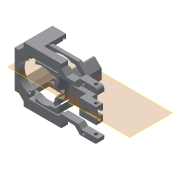
# Autodesk Inventor part: 20_focus_inlet_linearflexure_v0
Saved by Autodesk Inventor 2019.4 (Build 234330000, 330)
## iProperties
Created: 2020-02-03
Part Number: 20_focus_inlet_linearflexure_v0
Material: Generic
Document SubType Name: Modeling
Designer: diederichbenedict
Density: 1 g/cm^3
Appearance: Default
Author: diederichbenedict
Autodesk Inventor part; units mm, degrees
(part 1 of 2)
ref_plane "Work Plane1" through (0, 0, 0) normal (0, 0, 1) x (1, 0, 0)
sketch "Sketch1" plane through (0, 0, 0) normal (0, 0, 1) x (1, 0, 0)
  line L0 (33.5, -15.3849) -> (35.5, -15.3849) projected
  line L1 (35.5, -15.3849) -> (35.5, -14.1603) projected
  arc A0 (35.5, -14.1603) -> (35.3294, -13.8326) centre (35.1, -14.1603) ccw projected
  line L2 (35.3294, -13.8326) -> (34.0923, -12.9664) projected
  arc A1 (33.8775, -12.693) -> (34.0923, -12.9664) centre (34.4364, -12.4749) ccw projected
  arc A2 (33.8775, -12.693) -> (33.8775, -21.107) centre (23.1, -16.9) ccw projected
  arc A3 (34.0923, -20.8336) -> (33.8775, -21.107) centre (34.4364, -21.3251) ccw construction
  line L3 (34.0923, -20.8336) -> (35.3294, -19.9674) construction
  arc A4 (35.3294, -19.9674) -> (35.5, -19.6397) centre (35.1, -19.6397) ccw construction
  line L4 (35.5, -19.6397) -> (35.5, -18.4151) construction
  line L5 (35.5, -18.4151) -> (33.5, -18.4151) construction
  line L6 (33.5, -18.4151) -> (33.5, -15.3849) projected
  line L7 (30.0099, -20.9316) -> (30.0099, -25.4) construction
  line L8 (30.0099, -25.4) -> (27.6057, -25.4) construction
  line L9 (27.6057, -25.4) -> (27.6057, -23.5105) construction
  arc A5 (27.6057, -10.2895) -> (27.6057, -23.5105) centre (23.1, -16.9) ccw construction
  line L10 (27.6057, -10.2895) -> (27.6057, -8.4) construction
  line L11 (27.6057, -8.4) -> (30.0099, -8.4) construction
  line L12 (30.0099, -8.4) -> (30.0099, -12.8684) projected
  arc A6 (30.0099, -20.9316) -> (30.0099, -12.8684) centre (23.1, -16.9) ccw projected
  line L13 (23.1, -16.9) -> (97.1528, -16.9) construction
  arc A7 (31.4223, -8.5777) -> (34.0638, -21.1797) centre (23.1, -16.9) ccw
  arc A8 (34.0638, -12.6203) -> (34.207, -12.8025) centre (34.4364, -12.4749) ccw
  line L14 (34.207, -12.8025) -> (35.4441, -13.6688)
  arc A9 (35.7, -14.1603) -> (35.4441, -13.6688) centre (35.1, -14.1603) ccw
  line L15 (35.7, -14.1603) -> (35.7, -15.5849)
  line L16 (35.7, -15.5849) -> (33.7, -15.5849)
  line L17 (33.7, -15.5849) -> (33.7, -18.2151)
  line L18 (33.7, -18.2151) -> (35.7, -18.2151) construction
  line L19 (35.7, -18.2151) -> (35.7, -19.6397) construction
  arc A10 (35.4441, -20.1312) -> (35.7, -19.6397) centre (35.1, -19.6397) ccw construction
  line L20 (35.4441, -20.1312) -> (34.207, -20.9975) construction
  arc A11 (34.207, -20.9975) -> (34.0638, -21.1797) centre (34.4364, -21.3251) ccw construction
  circle A12 centre (33.6, -15.6849) radius 0.1 construction
  line L21 (35.7, -15.5849) -> (35.7, -16.9) construction
  line L22 (35.7, -15.5849) -> (35.7, -16.9)
  line L23 (23.1, -16.9) -> (31.4223, -8.5777)
  line L24 (23.1, -16.9) -> (34.8695, -16.9) construction
  line L25 (32.6022, -7.3978) -> (33.5436, -6.4564)
  line L26 (33.5436, -6.4564) -> (34.8883, -6.4564)
  line L27 (40.7, -12.2681) -> (40.7, -16.9)
  line L28 (35.7, -16.9) -> (40.7, -16.9)
  line L29 (35.7, -16.9) -> (39.7, -16.9)
  line L30 (39.7, -16.9) -> (39.7, -15.2)
  line L31 (39.7, -15.2) -> (35.7, -15.2)
  line L32 (35.7, -15.2) -> (35.7, -16.9)
  line L33 (39.7, -15.2) -> (36.7, -15.2)
  line L34 (36.7, -15.2) -> (36.7, -13.4)
  line L35 (36.7, -13.4) -> (39.7, -13.4)
  line L36 (39.7, -13.4) -> (39.7, -15.2)
  line L37 (33.5436, -6.4564) -> (34.8883, -6.4564) construction
  line L38 (40.7, -12.2681) -> (34.8883, -6.4564)
  line L39 (40.7, -12.2681) -> (48.919, -12.2681) construction
  arc A13 (34.0638, -12.6203) -> (32.6022, -7.3978) centre (18.0334, -14.2911) ccw
  point P0 (0, 0)
  dimension "d0" = 0.2
  dimension "d1" = 45
  dimension "d2" = 3
  dimension "d6" = 1.7
  dimension "d7" = 4
  dimension "d8" = 3.5
  dimension "d9" = 3
  dimension "d46" = 1
  dimension "d47" = 135
  constraints: 54 end point, 12 point on circle, 7 centre point, 7 horizontal, 4 parallel, 4 perpendicular, 3 point on line, 3 tangent, 2 collinear, 2 equal length, 10 other
  measures "d0" radial gap between concentric circles of A2 A7
  measures "d1" angle of L24 L23
  measures "d2" distance of L23.end L25.end
  measures "d6" distance of L30.end L29.end
  measures "d7" distance between parallel lines of L30 L21
  measures "d8" distance between parallel lines of L13 L35
  measures "d9" distance between parallel lines of L36 L34
  measures "d46" distance between parallel lines of L27 L30
  measures "d47" angle of L39 L38
extrude "Extrusion1" add sketch "Sketch1" against normal blind 35 contours A13 L25 L26 L38 L27 L28 L30 L36 L35 L34 L31 L15 A9 L14 A8
sketch "Sketch2" plane through (0, 0, 0) normal (0, 0, 1) x (1, 0, 0)
  line L0 (39.7, -13.4) -> (39.7, -16.9) projected
  line L1 (39.7, -16.9) -> (40.7, -16.9) projected
  line L2 (40.7, -16.9) -> (40.7, -12.2681) projected
  line L3 (33.5436, -6.4564) -> (32.6022, -7.3978) projected
  arc A0 (34.0638, -12.6203) -> (34.207, -12.8025) centre (34.4364, -12.4749) ccw projected
  line L4 (34.207, -12.8025) -> (35.4441, -13.6688) projected
  arc A1 (35.7, -14.1603) -> (35.4441, -13.6688) centre (35.1, -14.1603) ccw projected
  line L5 (35.7, -14.1603) -> (35.7, -15.2) projected
  line L6 (35.7, -15.2) -> (36.7, -15.2) projected
  line L7 (36.7, -15.2) -> (36.7, -13.4) projected
  line L8 (36.7, -13.4) -> (39.7, -13.4) projected
  line L9 (95.8, 0) -> (0, 0) projected
  line L10 (6, -33.8) -> (89.8, -33.8) projected
  line L11 (6, -33.8) -> (6, 0) projected
  line L12 (11, -0.7) -> (46, -0.7)
  line L13 (45.9987, -4.2) -> (45.9987, -4.7)
  line L14 (11, -4.3971) -> (11, -0.7)
  line L15 (45.9987, -4.7) -> (41.9987, -4.7)
  line L16 (42, -6.1887) -> (42, -16.9)
  line L17 (42, -16.9) -> (46, -16.9)
  line L18 (46, -16.9) -> (46, -10.1887)
  line L19 (6.2, -0.1) -> (10.2, -0.1)
  line L20 (10.2, -0.1) -> (10.2, -16.9)
  line L21 (10.2, -16.9) -> (6.2, -16.9)
  line L22 (6.2, -16.9) -> (6.2, -0.1)
  line L23 (46, -16.9) -> (61, -16.9)
  line L24 (61, -16.9) -> (61, -13.9)
  line L25 (61, -13.9) -> (46, -13.9)
  line L26 (46, -13.9) -> (46, -16.9)
  arc A2 (79.6921, -19.4) -> (79.6921, -14.4) centre (79.6921, -16.9) ccw projected
  line L27 (56, -10.9) -> (56, -13.9)
  line L28 (6.2, -0.1) -> (10.2, -0.1)
  line L29 (10.2, -0.1) -> (10.2, 4.9)
  line L30 (10.2, 4.9) -> (6.2, 4.9)
  line L31 (6.2, 4.9) -> (6.2, -0.1)
  line L32 (1.6162, -33.8) -> (1.6162, 0) projected
  line L33 (-2, 0) -> (1.6162, 0) projected
  line L34 (-2, -33.8) -> (-2, 0) projected
  line L35 (1.6162, -33.8) -> (-2, -33.8) projected
  line L36 (6.2, -16.9) -> (-2, -16.9)
  line L37 (-2, -16.9) -> (-2, -0.2)
  line L38 (-2, -0.2) -> (6.2, -0.2)
  line L39 (6.2, -0.2) -> (6.2, -16.9)
  line L40 (-2, 0) -> (0, 0) projected
  line L41 (10.2, 4.9) -> (89.6, 4.9)
  line L42 (89.6, 4.9) -> (89.6, 0)
  line L43 (89.6, 0) -> (10.2, 0)
  line L44 (10.2, 0) -> (10.2, 4.9)
  line L45 (89.8, 0) -> (89.8, 4.5) projected
  line L46 (95.8, 0) -> (89.8, 0) projected
  line L47 (97.8, -41.8) -> (97.8, 0) construction
  line L48 (94.1838, 0) -> (94.1838, -33.8) projected
  line L49 (97.8, -33.8) -> (94.1838, -33.8) projected
  line L50 (97.8, -33.8) -> (97.8, 0) projected
  line L51 (94.1838, 0) -> (97.8, 0) projected
  line L52 (97.8, -0.2) -> (85.8, -0.2)
  line L53 (85.8, -0.2) -> (85.8, -4.2)
  line L54 (85.8, -4.2) -> (97.8, -4.2)
  line L55 (97.8, -4.2) -> (97.8, -0.2)
  line L56 (85.8, -0.2) -> (89.6, -0.2)
  line L57 (89.6, -0.2) -> (89.6, 0)
  line L58 (89.6, 0) -> (85.8, 0)
  line L59 (85.8, 0) -> (85.8, -0.2)
  line L60 (40.7, -12.2681) -> (34.8883, -6.4564) projected
  line L61 (34.8883, -6.4564) -> (33.5436, -6.4564) projected
  line L62 (42, -12.2664) -> (34.1307, -4.3971)
  line L63 (42, -12.2664) -> (53.1289, -12.2664) construction
  line L64 (36.5113, -0.7) -> (46, -10.1887)
  line L65 (36.5113, -0.7) -> (49.9303, -0.7) construction
  line L66 (45.9987, -4.7) -> (41.9987, -4.7)
  line L67 (34.1307, -4.3971) -> (11, -4.3971)
  line L68 (97.8, -4.2) -> (94.1838, -4.2)
  line L69 (94.1838, -4.2) -> (94.1838, -16.9)
  line L70 (94.1838, -16.9) -> (97.8, -16.9)
  line L71 (97.8, -16.9) -> (97.8, -4.2)
  line L72 (61, -13.9) -> (56, -13.9)
  line L73 (56, -13.9) -> (56, -9.9)
  line L74 (56, -9.9) -> (61, -9.9)
  line L75 (61, -9.9) -> (61, -13.9)
  circle A3 centre (23.1, -16.9) radius 10 projected
  circle A4 centre (23.1, -16.9) radius 12.5 projected
  arc A5 (30.5468, -4.3971) -> (15.6532, -4.3971) centre (23.1, -16.9) ccw
  arc A6 (34.0638, -12.6203) -> (32.6022, -7.3978) centre (18.0334, -14.2911) ccw projected
  dimension "d10" = 35
  dimension "d11" = 4
  dimension "d12" = 5
  dimension "d13" = 0.7
  dimension "d14" = 4
  dimension "d15" = 4
  dimension "d16" = 0.2
  dimension "d17" = 15
  dimension "d18" = 3
  dimension "d25" = 5
  dimension "d28" = 0.1
  dimension "d29" = 5
  dimension "d30" = 0.2
  dimension "d31" = 0.2
  dimension "d32" = 12
  dimension "d33" = 4
  dimension "d34" = 0.2
  dimension "d48" = 135
  dimension "d49" = 45
  dimension "d59" = 1.3
  dimension "d68" = 7
  constraints: 100 end point, 23 parallel, 13 horizontal, 11 perpendicular, 11 point on line, 2 equal length, 2 point on circle, 1 centre point, 1 coincident, 1 midpoint
  measures "d10" distance of L13.end L14.start
  measures "d11" distance of L12.end L13.end
  measures "d12" distance between parallel lines of L14 L11
  measures "d13" distance between parallel lines of L12 L9
  measures "d14" distance of L17.end L16.end
  measures "d15" distance of L20.end L21.end
  measures "d16" distance between parallel lines of L22 L11
  measures "d17" distance of L25.end L24.end
  measures "d18" distance of L24.end L23.end
  measures "d25" distance between parallel lines of L24 L27
  measures "d28" distance between parallel lines of L9 L19
  measures "d29" distance of L29.end L28.end
  measures "d30" distance between parallel lines of L38 L40
  measures "d31" distance between parallel lines of L45 L42
  measures "d32" distance of L54.end L53.end
  measures "d33" distance of L53.end L52.end
  measures "d34" distance between parallel lines of L9 L52
  measures "d48" angle of L63 L62
  measures "d49" angle of L64 L65
  measures "d59" distance between parallel lines of L16 L2
  measures "d68" distance between parallel lines of L74 L23
extrude "Extrusion2" add sketch "Sketch2" against normal blind 6 contours L52 L50 L54 L48 | L48 L54 L53 L52 | L57 L52 L59 L9 | L9 L29 L41 L42 | L54 L50 L70 L48 | L29 L19 L31 L9 | L9 L31 L30 L29 | L20 L21 L22 L19 | L38 L22 L36 L11 | L11 L36 L32 L38 | L32 L36 L34 L38 | L12 L64 L16 L62 L67 A5 L14 | L64 L18 L17 L16 | L25 L24 L23 L18 | L27 L73 L74 L75 L25
sketch "Sketch3" plane through (0, 0, -6) normal (0, 0, 1) x (1, 0, 0)
  line L0 (42, -12.2664) -> (42, -16.9) projected
  line L1 (42, -16.9) -> (61, -16.9) projected
  line L2 (61, -16.9) -> (61, -9.9) projected
  line L3 (56, -13.9) -> (46, -13.9) projected
  line L4 (36.5113, -0.7) -> (11, -0.7) projected
  line L5 (11, -0.7) -> (11, -4.3971) projected
  line L6 (39.7, -13.4) -> (39.7, -16.9) projected
  line L7 (39.7, -16.9) -> (40.7, -16.9) projected
  line L8 (40.7, -16.9) -> (40.7, -12.2681) projected
  line L9 (33.5436, -6.4564) -> (32.6022, -7.3978) projected
  arc A0 (34.0638, -12.6203) -> (34.207, -12.8025) centre (34.4364, -12.4749) ccw projected
  line L10 (34.207, -12.8025) -> (35.4441, -13.6688) projected
  arc A1 (35.7, -14.1603) -> (35.4441, -13.6688) centre (35.1, -14.1603) ccw projected
  line L11 (35.7, -14.1603) -> (35.7, -15.2) projected
  line L12 (35.7, -15.2) -> (36.7, -15.2) projected
  line L13 (36.7, -15.2) -> (36.7, -13.4) projected
  line L14 (36.7, -13.4) -> (39.7, -13.4) projected
  line L15 (6.2, 4.9) -> (6.2, -0.2) projected
  line L16 (-2, -16.9) -> (10.2, -16.9) projected
  line L17 (10.2, -16.9) -> (10.2, 0) projected
  line L18 (11, -4.3971) -> (11, -0.7) projected
  line L19 (10.2, 0) -> (10.2, -16.9) projected
  line L20 (11, -0.7) -> (10.2, -0.7)
  line L21 (10.2, -0.7) -> (10.2, -4.3971)
  line L22 (10.2, -4.3971) -> (11, -4.3971)
  line L23 (11, -4.3971) -> (11, -0.7)
  line L24 (42, -16.9) -> (42, -12.2664) projected
  line L25 (40.7, -16.9) -> (42, -16.9)
  line L26 (42, -16.9) -> (42, -6.4564)
  line L27 (42, -6.4564) -> (40.7, -6.4564)
  line L28 (40.7, -6.4564) -> (40.7, -16.9)
  line L29 (6.2, -0.2) -> (-2, -0.2) projected
  line L30 (-2, -0.2) -> (-2, -16.9) projected
  line L31 (89.6, 4.9) -> (6.2, 4.9) projected
  line L32 (10.2, 0) -> (85.8, 0) projected
  line L33 (89.6, -0.2) -> (89.6, 4.9) projected
  line L34 (85.8, 0) -> (85.8, -4.2) projected
  line L35 (85.8, -4.2) -> (94.1838, -4.2) projected
  line L36 (97.8, -16.9) -> (97.8, -0.2) projected
  line L37 (97.8, -0.2) -> (89.6, -0.2) projected
  line L38 (40.7, -12.2681) -> (34.8883, -6.4564) projected
  line L39 (34.8883, -6.4564) -> (33.5436, -6.4564) projected
  line L40 (46, -13.9) -> (46, -10.1887) projected
  line L41 (46, -10.1887) -> (36.5113, -0.7) projected
  line L42 (30.5468, -4.3971) -> (34.1307, -4.3971) projected
  line L43 (34.1307, -4.3971) -> (42, -12.2664) projected
  line L44 (94.1838, -4.2) -> (94.1838, -16.9) projected
  line L45 (94.1838, -16.9) -> (97.8, -16.9) projected
  line L46 (61, -9.9) -> (56, -9.9) projected
  line L47 (56, -9.9) -> (56, -13.9) projected
  line L48 (11, -4.3971) -> (15.6532, -4.3971) projected
  arc A2 (30.5468, -4.3971) -> (15.6532, -4.3971) centre (23.1, -16.9) ccw projected
  arc A3 (34.0638, -12.6203) -> (32.6022, -7.3978) centre (18.0334, -14.2911) ccw projected
  point P0 (0, 0)
  point P1 (42, -4.4)
  point P2 (10.2, -0.1)
  point P3 (10.2, 4.9)
  constraints: 16 end point, 4 parallel, 2 horizontal, 2 perpendicular, 2 point on line
extrude "Extrusion3" add sketch "Sketch3" along normal blind 0.5 contours L43 L28 L27 L26 | L0 L25 L8 L28 L43 | L22 L17 L20 L5
sketch "Sketch5" plane through (0, 0, -6) normal (0, 0, -1) x (-1, 0, 0)
  line L0 (2, -16.9) -> (2, -0.2) projected
  line L1 (2, -0.2) -> (-6.2, -0.2) projected
  line L2 (-6.2, -0.2) -> (-6.2, 4.9) projected
  line L3 (-6.2, 4.9) -> (-89.6, 4.9) projected
  line L4 (-89.6, 4.9) -> (-89.6, -0.2) projected
  line L5 (-89.6, -0.2) -> (-97.8, -0.2) projected
  line L6 (-97.8, -0.2) -> (-97.8, -16.9) projected
  line L7 (-94.1838, -4.2) -> (-85.8, -4.2) projected
  line L8 (-85.8, -4.2) -> (-85.8, 0) projected
  line L9 (-85.8, 0) -> (-10.2, 0) projected
  line L10 (-10.2, -4.3971) -> (-10.2, -16.9) projected
  line L11 (-10.2, -16.9) -> (2, -16.9) projected
  line L12 (-97.8, -16.9) -> (-94.1838, -16.9) projected
  line L13 (-94.1838, -16.9) -> (-94.1838, -4.2) projected
  line L14 (-10.2, -4.3971) -> (-10.2, -0.7) projected
  arc A0 (-1, -16.9) -> (-10.2, -4.3971) centre (-14.0958, -16.9) ccw
  line L15 (-10.2, 0) -> (-10.2, -0.7) projected
  line L16 (-36.5113, -0.7) -> (-10.2, -0.7) projected
  line L17 (-36.5113, -0.7) -> (-46, -10.1887) projected
  line L18 (-46, -10.1887) -> (-46, -13.9) projected
  line L19 (-46, -13.9) -> (-56, -13.9) projected
  line L20 (-56, -13.9) -> (-56, -9.9) projected
  line L21 (-56, -9.9) -> (-61, -9.9) projected
  line L22 (-61, -9.9) -> (-61, -16.9) projected
  line L23 (-61, -16.9) -> (-40.7, -16.9) projected
  line L24 (-40.7, -12.2681) -> (-40.7, -16.9) projected
  line L25 (-40.7, -10.9664) -> (-40.7, -12.2681) projected
  line L26 (-40.7, -10.9664) -> (-34.1307, -4.3971) projected
  line L27 (-34.1307, -4.3971) -> (-30.5468, -4.3971) projected
  arc A1 (-15.6532, -4.3971) -> (-30.5468, -4.3971) centre (-23.1, -16.9) ccw projected
  line L28 (-15.6532, -4.3971) -> (-10.2, -4.3971) projected
  dimension "d65" = 0
  dimension "d66" = 3
  constraints: 2 point on circle, 1 centre point, 1 point on line
  measures "d65" distance from line of A0.centre L11
  measures "d66" distance from line of L0 A0.start
extrude "Extrusion5" cut sketch "Sketch5" against normal through all contours L11 L10 A0
sketch "Sketch6" plane through (0, 0, -6) normal (0, 0, -1) x (-1, 0, 0)
  line L0 (-46, -13.9) -> (-56, -13.9) projected
  line L1 (-61, -9.9) -> (-61, -16.9) projected
  line L2 (-10.2, -16.9) -> (2, -16.9) construction
  line L3 (-10.2, -4.3971) -> (-10.2, -16.9) projected
  line L4 (2, -0.2) -> (2, -16.9) projected
  line L5 (2, -0.2) -> (-10.2, -0.2)
  line L6 (2, -4.4) -> (2, -0.2)
  line L7 (2, -4.4) -> (2, -0.2) construction
  line L8 (2, -0.2) -> (-10.2, -0.2) construction
  line L9 (-36.5113, -0.7) -> (-46, -10.1887) projected
  line L10 (-46, -10.1887) -> (-46, -13.9) projected
  line L11 (-40.7, -10.9664) -> (-34.1307, -4.3971) projected
  line L12 (-56, -13.9) -> (-56, -9.9) projected
  line L13 (-56, -9.9) -> (-61, -9.9) projected
  line L14 (2, -4.4) -> (-10.2, -4.4)
  line L15 (-10.2, -4.4) -> (-10.2, -0.2)
  line L16 (-10.2, -0.2) -> (2, -0.2)
  line L17 (2, -0.2) -> (2, -4.4)
  line L18 (-34.1307, -4.3971) -> (-30.5468, -4.3971) projected
  arc A0 (-15.6532, -4.3971) -> (-30.5468, -4.3971) centre (-23.1, -16.9) ccw projected
  line L19 (-40.7, -10.9664) -> (-40.7, -12.2681) projected
  line L20 (-36.5113, -0.7) -> (-10.2, -0.7) projected
  line L21 (-61, -16.9) -> (-40.7, -16.9) projected
  line L22 (-40.7, -12.2681) -> (-40.7, -16.9) projected
  line L23 (-15.6532, -4.3971) -> (-10.2, -4.3971) projected
  line L24 (2, -16.9) -> (2, -0.2) projected
  line L25 (2, -0.2) -> (-6.2, -0.2) projected
  line L26 (-6.2, -0.2) -> (-6.2, 4.9) projected
  line L27 (-6.2, 4.9) -> (-89.6, 4.9) projected
  line L28 (-89.6, 4.9) -> (-89.6, -0.2) projected
  line L29 (-89.6, -0.2) -> (-97.8, -0.2) projected
  line L30 (-97.8, -0.2) -> (-97.8, -16.9) projected
  line L31 (-97.8, -16.9) -> (-94.1838, -16.9) projected
  line L32 (-94.1838, -16.9) -> (-94.1838, -4.2) projected
  line L33 (-94.1838, -4.2) -> (-85.8, -4.2) projected
  line L34 (-85.8, -4.2) -> (-85.8, 0) projected
  line L35 (-85.8, 0) -> (-10.2, 0) projected
  line L36 (-10.2, 0) -> (-10.2, -0.7) projected
  line L37 (-10.2, -4.3971) -> (-10.2, -16.9) projected
  line L38 (-10.2, -16.9) -> (2, -16.9) projected
  line L39 (2, -16.9) -> (2, -0.2) projected
  line L40 (2, -0.2) -> (-6.2, -0.2) projected
  line L41 (-6.2, -0.2) -> (-6.2, 4.9) projected
  line L42 (-6.2, 4.9) -> (-89.6, 4.9) projected
  line L43 (-89.6, 4.9) -> (-89.6, -0.2) projected
  line L44 (-89.6, -0.2) -> (-97.8, -0.2) projected
  line L45 (-97.8, -0.2) -> (-97.8, -16.9) projected
  line L46 (-97.8, -16.9) -> (-94.1838, -16.9) projected
  line L47 (-94.1838, -16.9) -> (-94.1838, -4.2) projected
  line L48 (-94.1838, -4.2) -> (-85.8, -4.2) projected
  line L49 (-85.8, -4.2) -> (-85.8, 0) projected
  line L50 (-85.8, 0) -> (-10.2, 0) projected
  line L51 (-10.2, 0) -> (-10.2, -0.7) projected
  line L52 (-36.5113, -0.7) -> (-10.2, -0.7) projected
  line L53 (-36.5113, -0.7) -> (-46, -10.1887) projected
  line L54 (-46, -10.1887) -> (-46, -13.9) projected
  line L55 (-46, -13.9) -> (-56, -13.9) projected
  line L56 (-56, -13.9) -> (-56, -9.9) projected
  line L57 (-56, -9.9) -> (-61, -9.9) projected
  line L58 (-61, -9.9) -> (-61, -16.9) projected
  line L59 (-61, -16.9) -> (-40.7, -16.9) projected
  line L60 (-40.7, -12.2681) -> (-40.7, -16.9) projected
  line L61 (-40.7, -10.9664) -> (-40.7, -12.2681) projected
  line L62 (-40.7, -10.9664) -> (-34.1307, -4.3971) projected
  line L63 (-34.1307, -4.3971) -> (-30.5468, -4.3971) projected
  arc A1 (-15.6532, -4.3971) -> (-30.5468, -4.3971) centre (-23.1, -16.9) ccw projected
  line L64 (-15.6532, -4.3971) -> (-10.2, -4.3971) projected
  point P0 (0, 0)
  constraints: 16 end point, 2 horizontal, 2 parallel, 1 perpendicular
ref_plane "Work Plane2" through (6, 4.5, -33.8) normal (0, 0, 1) x (1, 0, 0)
extrude "Extrusion6" add sketch "Sketch6" along normal up to surface (27.8 mm away) contours L15 L5 L4 L14 L3
ref_plane "Work Plane3" through (0, 0, -18) normal (0, 0, -1) x (-1, 0, 0)
sketch "Sketch7" plane through (0, 0, -18) normal (0, 0, -1) x (-1, 0, 0)
  line L0 (-11, -0.7) -> (-10.2, -0.7) projected
  line L1 (-10.2, -4.3971) -> (-11, -4.3971) projected
  line L2 (-11.9304, -0.7) -> (-11, -0.7) projected
  line L3 (-11.9304, -4.3971) -> (-11.9304, -0.7) projected
  line L4 (-46, -13.9) -> (-56, -13.9) projected
  line L5 (-61, -9.9) -> (-61, -16.9) projected
  line L6 (-40.7, -16.9) -> (-42, -16.9) projected
  line L7 (-40.7, -16.9) -> (-40.7, -12.2681) projected
  line L8 (-10.2, -0.2) -> (-10.2, -4.4) projected
  line L9 (2, -4.4) -> (2, -0.2) projected
  line L10 (2, -0.2) -> (-10.2, -0.2) projected
  line L11 (-46, -13.9) -> (-46, -16.9)
  line L12 (-61, -16.9) -> (-42, -16.9) projected
  line L13 (-40.7, -10.9664) -> (-40.7, -12.2681) projected
  line L14 (-36.5113, -0.7) -> (-46, -10.1887) projected
  line L15 (-46, -10.1887) -> (-46, -13.9) projected
  line L16 (-40.7, -10.9664) -> (-34.1307, -4.3971) projected
  line L17 (-11, -4.3971) -> (-11.9304, -4.3971) projected
  line L18 (-46, -13.9) -> (-46, -16.9)
  line L19 (-56, -13.9) -> (-56, -9.9) projected
  line L20 (-56, -9.9) -> (-61, -9.9) projected
  line L21 (-10.2, -4.4) -> (2, -4.4) projected
  line L22 (-34.1307, -4.3971) -> (-30.5468, -4.3971) projected
  arc A0 (-15.6532, -4.3971) -> (-30.5468, -4.3971) centre (-23.1, -16.9) ccw projected
  line L23 (-11, -0.7) -> (-11, -4.3971) projected
  line L24 (-40.7, -10.9664) -> (-40.7, -12.2681) projected
  line L25 (-40.7, -10.9664) -> (-42, -12.2664) projected
  line L26 (-42, -12.2664) -> (-42, -16.9) projected
  line L27 (-36.5113, -0.7) -> (-10.2, -0.7) projected
  line L28 (-61, -16.9) -> (-40.7, -16.9) projected
  line L29 (-40.7, -12.2681) -> (-40.7, -16.9) projected
  line L30 (-15.6532, -4.3971) -> (-10.2, -4.3971) projected
  line L31 (-11, -0.7) -> (-11, -4.3971) projected
  line L32 (-10.2, -4.3971) -> (-10.2, -0.7) projected
  line L33 (-10.2, -4.3971) -> (-10.2, -0.7) projected
  point P0 (0, 0)
  constraints: 4 end point, 1 collinear, 1 point on line
extrude "Extrusion7" add sketch "Sketch7" along normal blind 3 contours L23 L17 L3 L2 | L3 L30 A0 L22 L16 L25 L26 L12 L11 L15 L14 L27
sketch "Sketch8" plane through (0, 0, -18) normal (0, 0, 1) x (1, 0, 0)
  line L0 (11, -0.7) -> (10.2, -0.7) projected
  line L1 (10.2, -4.3971) -> (11, -4.3971) projected
  line L2 (40.7, -16.9) -> (42, -16.9) projected
  line L3 (40.7, -16.9) -> (40.7, -12.2681) projected
  line L4 (40.7, -10.9664) -> (40.7, -12.2681) projected
  line L5 (40.7, -10.9664) -> (42, -12.2664) projected
  line L6 (42, -12.2664) -> (42, -16.9) projected
  line L7 (11, -0.7) -> (11, -4.3971) projected
  line L8 (10.2, -4.3971) -> (10.2, -0.7) projected
  point P0 (0, 0)
  point P1 (10.2, -4.4)
extrude "Extrusion8" add sketch "Sketch8" against normal blind 0.5
sketch "Sketch9" plane through (10.2, -0.7, -18) normal (0, 1, 0) x (1, 0, 0)
  line L0 (26.3113, 0) -> (0, 0) projected
  line L1 (26.3113, 0) -> (26.3113, 3) projected
  line L2 (0, 3) -> (26.3113, 3) projected
  line L3 (0, 0) -> (0, 3) projected
  line L4 (0.8, 0.5) -> (0, 0.5) projected
  line L5 (0.8, 0.5) -> (1.8167, 3)
  line L6 (23.9307, 3) -> (0.8, 3) projected
  line L7 (0.8, 3) -> (1.8167, 3)
  line L8 (0.8, 3) -> (0.8, 0.5)
  point P0 (-10.2, -18)
  constraints: 6 end point, 1 collinear, 1 point on line
extrude "Extrusion9" cut sketch "Sketch9" against normal up to surface (3.6971 mm away) contours L8 L2 L5
sketch "Sketch10" plane through (0, 0, -6) normal (0, 0, -1) x (-1, 0, 0)
  arc A0 (-75.8, -1.5) -> (-75.8, 2.7) centre (-75.8, 0.6) ccw projected
  line L0 (-10.2, 0) -> (-10.2, -0.2) projected
  line L1 (-89.6, 4.9) -> (-72.3075, 4.9)
  line L2 (-72.3075, 4.9) -> (-72.3075, -2.4765)
  line L3 (-72.3075, -2.4765) -> (-89.6, -2.4765)
  line L4 (-89.6, -2.4765) -> (-89.6, 4.9)
  line L5 (-10.2, -16.9) -> (2, -16.9) projected
  line L6 (2, -4.4) -> (-10.2, -4.4) projected
  line L7 (-10.2, -0.2) -> (-6.2, -0.2) projected
  line L8 (-6.2, -0.2) -> (-6.2, 4.9) projected
  line L9 (-6.2, 4.9) -> (-89.6, 4.9) projected
  line L10 (-89.6, 4.9) -> (-89.6, -0.2) projected
  line L11 (-89.6, -0.2) -> (-97.8, -0.2) projected
  line L12 (-97.8, -0.2) -> (-97.8, -16.9) projected
  line L13 (-97.8, -16.9) -> (-94.1838, -16.9) projected
  line L14 (-94.1838, -16.9) -> (-94.1838, -4.2) projected
  line L15 (-94.1838, -4.2) -> (-85.8, -4.2) projected
  line L16 (-85.8, -4.2) -> (-85.8, 0) projected
  line L17 (-85.8, 0) -> (-10.2, 0) projected
  line L18 (-10.2, -4.4) -> (-10.2, -16.9) projected
  line L19 (2, -16.9) -> (2, -4.4) projected
  point P0 (0, 0)
  constraints: 8 end point, 2 parallel, 1 horizontal, 1 perpendicular
ref_plane "Work Plane4" through (10.2, -4.4, -20.3) normal (0, 0, -1) x (-1, 0, 0)
extrude "Extrusion10" add sketch "Sketch10" along normal up to surface (14.3 mm away) contours L17 L16 L3 L4 L1 L2 | L2 L3 L16 L17
sketch "Sketch11" plane through (89.6, 4.9, -20.3) normal (0, 0, -1) x (-1, 0, 0)
  arc A0 (13.8, -6.4) -> (13.8, -2.2) centre (13.8, -4.3) ccw projected
  circle A1 centre (13.8, -4.3) radius 1.4
  point P0 (89.6, -4.9)
  dimension "d54" = 2.8
  constraints: 1 centre point, 1 coincident
  measures "d54" diameter of A1
extrude "Extrusion11" cut sketch "Sketch11" against normal through all
sketch "Sketch13" plane through (61, -16.9, 0) normal (1, 0, 0) x (0, 0, -1)
  line L0 (0, 3) -> (6, 3) projected
  line L1 (6, 0) -> (6, 4.6336) projected
  line L2 (0, 0) -> (35, 0) projected
  line L3 (21, 0) -> (18, 0) projected
  line L4 (0, 4.6319) -> (0, 10.4436) projected
  line L5 (0, 10.4436) -> (0, 9.5022) projected
  line L6 (0, 4.2797) -> (0, 4.0975) projected
  line L7 (0, 4.0975) -> (0, 3.2312) projected
  line L8 (0, 3.2312) -> (0, 2.7397) projected
  line L9 (0, 2.7397) -> (0, 1.7) projected
  line L10 (0, 1.7) -> (0, 3.5) projected
  line L11 (0, 3.5) -> (0, 0) projected
  line L12 (0, 0) -> (6, 0) projected
  line L13 (6, 0) -> (0, 0)
  line L14 (0, 0) -> (0, 1.7)
  line L15 (0, 1.7) -> (6, 1.7)
  line L16 (6, 1.7) -> (6, 0)
  line L17 (35, 1.7) -> (0, 1.7) projected
  line L18 (4.864, 1.7) -> (1.364, 1.7)
  line L19 (1.364, 1.7) -> (1.364, 4.55)
  line L20 (1.364, 4.55) -> (4.864, 4.55)
  line L21 (4.864, 4.55) -> (4.864, 1.7)
  line L22 (6, 1.7) -> (4.364, 1.7)
  line L23 (4.364, 1.7) -> (4.364, 7)
  line L24 (4.364, 7) -> (6, 7)
  line L25 (6, 7) -> (6, 1.7)
  line L26 (1.364, 4.55) -> (4.364, 4.55)
  line L27 (4.364, 4.55) -> (4.364, 7)
  line L28 (4.364, 7) -> (1.364, 7)
  line L29 (1.364, 7) -> (1.364, 4.55)
  line L30 (1.364, 7) -> (0, 7)
  line L31 (0, 7) -> (0, 1.7)
  line L32 (0, 1.7) -> (1.364, 1.7)
  line L33 (1.364, 1.7) -> (1.364, 7)
  line L34 (0, 3) -> (6, 3) projected
  line L35 (0, 9.5022) -> (0, 4.2797) projected
  line L36 (0, 0) -> (0, 4.6319) projected
  line L37 (18.5, 0) -> (35, 0) projected
  line L38 (6, 0) -> (18, 0) projected
  line L39 (0, 0) -> (6, 0) projected
  line L40 (0, 0) -> (5.5, 0) projected
  line L41 (0, 0) -> (5.5, 0) projected
  line L42 (18.5, 0) -> (21, 0) projected
  point P0 (0, 16.9)
  point P1 (6, 3)
  point P2 (6.5, 0)
  point P3 (0.5, 0)
  point P4 (0, 0)
  point P5 (0, 0)
  point P6 (0, 0)
  point P7 (0, 18.6)
  point P8 (0, 21.4)
  point P9 (0, 18.6)
  point P10 (0, 21.4)
  dimension "d60" = 1.7
  dimension "d61" = 3.5
  dimension "d62" = 2.85
  constraints: 40 end point, 10 parallel, 5 horizontal, 5 perpendicular, 1 point on line, 1 other
  measures "d60" distance of L13.end L10.start
  measures "d61" distance of L19.end L20.end
  measures "d62" distance of L18.end L19.end
extrude "Extrusion13" add sketch "Sketch13" along normal blind 10 contours L8 L7 L6 L31 L4 L30 L29 L19 L0 | L0 L19 L15 L9 L8 | L23 L20 L21 L0 | L0 L21 L15 L23 | L29 L28 L23 L20 | L21 L20 L23 L24 L25 L1 L0 | L0 L1 L15 L21
mirror "Mirror1" about plane through (6.2, -16.9, 0) normal (0, -1, 0) of "Extrusion1", "Extrusion2", "Extrusion3", "Extrusion5", "Extrusion6", "Extrusion7", "Extrusion8", "Extrusion9", "Extrusion10", "Extrusion11", "Extrusion13"
sketch "Sketch14" plane through (56, -9.9, 0) normal (0, 1, 0) x (1, 0, 0)
  line L0 (9.3, 20.8) -> (9.3, 18.3)
  line L1 (33.6, 0) -> (-49.8, 0) projected
  line L2 (33.6, 0) -> (33.6, 20.3) projected
  line L3 (33.6, 20.3) -> (16.3075, 20.3) projected
  line L4 (16.3075, 6) -> (16.3075, 20.3) projected
  line L5 (-49.8, 6) -> (16.3075, 6) projected
  line L6 (-49.8, 0) -> (-49.8, 6) projected
  circle A0 centre (11.813, 3) radius 1.45
  point P0 (-56, 0)
  point P1 (14.3156, 19.0518)
  dimension "d69" = 2.9
  constraints: 2 end point, 1 centre point, 1 vertical, 3 other
  measures "d69" diameter of A0
extrude "Extrusion14" cut sketch "Sketch14" along normal through all both and the other way through all contours A0
sketch "Sketch15" plane through (89.6, 4.9, -20.3) normal (0, 0, -1) x (-1, 0, 0)
  circle A0 centre (13.8, -4.3) radius 1.4 projected
  line L0 (0, 0) -> (17.2925, 0) projected
  line L1 (0, -7.3765) -> (0, 0) projected
  line L2 (17.2925, -7.3765) -> (0, -7.3765) projected
  line L3 (17.2925, 0) -> (17.2925, -7.3765) projected
  line L4 (-0.2, -38.7) -> (83.6, -38.7) projected
  circle A1 centre (13.8, -39.3) radius 1.4 projected
  line L5 (0, -43.6) -> (17.2925, -43.6) projected
  line L6 (17.2925, -43.6) -> (17.2925, -36.2235) projected
  line L7 (17.2925, -36.2235) -> (0, -36.2235) projected
  line L8 (0, -36.2235) -> (0, -43.6) projected
  line L9 (0, -36.2235) -> (3.8, -36.2235) projected
  line L10 (0, -43.6) -> (17.2925, -43.6) projected
  line L11 (0, -36.2235) -> (6, -36.2235)
  line L12 (6, -36.2235) -> (6, -43.6)
  line L13 (6, -43.6) -> (0, -43.6)
  line L14 (0, -43.6) -> (0, -36.2235)
  line L15 (0, 0) -> (17.2925, 0) projected
  line L16 (0, -7.3765) -> (6, -7.3765)
  line L17 (6, -7.3765) -> (6, 0)
  line L18 (6, 0) -> (0, 0)
  line L19 (0, 0) -> (0, -7.3765)
  point P0 (89.6, -4.9)
  dimension "d72" = 6
  constraints: 16 end point, 4 parallel, 3 point on line, 2 horizontal, 2 perpendicular
  measures "d72" distance of L12.end L13.end
extrude "Extrusion15" add sketch "Sketch15" along normal up to surface (13.5 mm away) contours L0 L17 L2 L1 | L8 L7 L12 L4 | L4 L12 L5 L8
sketch "Sketch16" plane through (0, 0, -6) normal (0, 0, -1) x (-1, 0, 0)
  line L0 (-10.1907, -29.4) -> (2, -29.4) construction
  line L1 (2, -4.4) -> (-10.1907, -4.4) construction
  line L2 (-10.1907, -4.4) -> (2, -4.4)
  line L3 (-10.1907, -29.4) -> (2, -29.4)
  line L4 (2, -29.4) -> (2, -27.4)
  line L5 (2, -33.6) -> (2, -33.6) projected
  line L6 (2, -27.4) -> (-6.2696, -27.4)
  arc A0 (-10.2, -29.4029) -> (-10.2, -4.3971) centre (-14.0958, -16.9) ccw projected
  line L7 (2, -4.4) -> (2, -6.4)
  line L8 (2, -6.4) -> (-6.2696, -6.4)
  arc A1 (-10.1907, -29.4) -> (-6.2696, -27.4) centre (-14.0958, -16.9) ccw
  arc A2 (-6.2696, -6.4) -> (-10.1907, -4.4) centre (-14.0958, -16.9) ccw
  line L9 (-10.2, -4.3971) -> (-10.2, -0.7) projected
  line L10 (2, -4.4) -> (2, -29.4) projected
  line L11 (-72.3075, 4.9) -> (-72.3075, 0) projected
  line L12 (-72.3075, 0) -> (-10.2, 0) projected
  line L13 (-10.2, 0) -> (-10.2, -0.2) projected
  line L14 (-10.2, -0.2) -> (-6.2, -0.2) projected
  line L15 (-6.2, -0.2) -> (-6.2, 4.9) projected
  line L16 (-6.2, 4.9) -> (-72.3075, 4.9) projected
  arc A3 (-10.1907, -29.4) -> (-10.1907, -4.4) centre (-14.0958, -16.9) ccw projected
  line L17 (-10.2, -33.1) -> (-10.2, -29.4029) projected
  line L18 (-10.2, -29.4029) -> (-15.6532, -29.4029) projected
  arc A4 (-15.6532, -29.4029) -> (-30.5468, -29.4029) centre (-23.1, -16.9) ccw projected
  line L19 (-34.1307, -29.4029) -> (-30.5468, -29.4029) projected
  line L20 (-40.7, -22.8336) -> (-34.1307, -29.4029) projected
  line L21 (-40.7, -22.8336) -> (-40.7, -21.5319) projected
  line L22 (-40.7, -12.2681) -> (-40.7, -21.5319) projected
  line L23 (-40.7, -10.9664) -> (-40.7, -12.2681) projected
  line L24 (-40.7, -10.9664) -> (-34.1307, -4.3971) projected
  line L25 (-34.1307, -4.3971) -> (-30.5468, -4.3971) projected
  arc A5 (-15.6532, -4.3971) -> (-30.5468, -4.3971) centre (-23.1, -16.9) ccw projected
  line L26 (-15.6532, -4.3971) -> (-10.2, -4.3971) projected
  line L27 (-36.5113, -0.7) -> (-10.2, -0.7) projected
  line L28 (-36.5113, -0.7) -> (-46, -10.1887) projected
  line L29 (-46, -10.1887) -> (-46, -13.9) projected
  line L30 (-46, -13.9) -> (-56, -13.9) projected
  line L31 (-56, -13.9) -> (-56, -9.9) projected
  line L32 (-56, -9.9) -> (-71, -9.9) projected
  line L33 (-71, -15.2) -> (-71, -9.9) projected
  line L34 (-61, -15.2) -> (-71, -15.2) projected
  line L35 (-61, -15.2) -> (-61, -18.6) projected
  line L36 (-61, -18.6) -> (-71, -18.6) projected
  line L37 (-71, -18.6) -> (-71, -23.9) projected
  line L38 (-56, -23.9) -> (-71, -23.9) projected
  line L39 (-56, -19.9) -> (-56, -23.9) projected
  line L40 (-46, -19.9) -> (-56, -19.9) projected
  line L41 (-46, -23.6113) -> (-46, -19.9) projected
  line L42 (-36.5113, -33.1) -> (-46, -23.6113) projected
  line L43 (-10.2, -33.1) -> (-36.5113, -33.1) projected
  line L44 (-72.3075, -33.8) -> (-72.3075, -38.7) projected
  line L45 (-6.2, -38.7) -> (-72.3075, -38.7) projected
  line L46 (-6.2, -33.6) -> (-6.2, -38.7) projected
  line L47 (-6.2, -33.6) -> (-10.2, -33.6) projected
  line L48 (-10.2, -33.8) -> (-10.2, -33.6) projected
  line L49 (-72.3075, -33.8) -> (-10.2, -33.8) projected
  point P0 (0, 0)
  point P1 (2, -0.2)
  dimension "d76" = 2
  dimension "d77" = 2
  constraints: 12 end point, 5 point on circle, 2 centre point, 2 concentric, 2 perpendicular, 2 other
  measures "d76" distance of L3.end L4.end
  measures "d77" distance of L2.end L7.end
extrude "Extrusion16" add sketch "Sketch16" along normal up to surface (27.8 mm away) contours L2 L7 L8 A0 | L6 L4 L3 A0
sketch "Sketch17" plane through (-2, -0.2, -33.8) normal (-1, 0, 0) x (0, 0, 1)
  line L0 (33.8, 0) -> (0, 0) construction
  line L1 (0, -6.2) -> (0, 0) construction
  line L2 (27.8, -6.2) -> (0, -6.2) construction
  line L3 (27.8, -6.2) -> (27.8, -27.2) construction
  line L4 (27.8, -27.2) -> (0, -27.2) construction
  line L5 (0, -27.2) -> (0, -33.4) construction
  line L6 (33.8, -33.4) -> (0, -33.4) construction
  line L7 (32.15, -3.5) -> (1.65, -3.5) construction
  line L8 (1.65, -3.5) -> (1.65, -29.9) construction
  line L9 (1.65, -29.9) -> (32.15, -29.9) construction
  line L10 (32.15, -29.9) -> (32.15, -3.5) construction
  line L11 (32.15, -3.5) -> (1.65, -29.9) construction
  line L12 (1.65, -3.5) -> (32.15, -29.9) construction
  circle A0 centre (1.65, -29.9) radius 1.5 construction
  circle A1 centre (1.65, -3.5) radius 1.5 construction
  circle A2 centre (32.15, -3.5) radius 1.5 construction
  circle A3 centre (32.15, -29.9) radius 1.5 construction
  circle A4 centre (1.65, -29.9) radius 1.2
  circle A5 centre (1.65, -3.5) radius 1.2
  circle A6 centre (32.15, -29.9) radius 1.2
  circle A7 centre (32.15, -3.5) radius 1.2
  line L13 (33.8, 0) -> (33.8, -33.4) projected
  point P0 (33.8, 0.2)
  point P1 (16.9, -16.7)
  dimension "d80" = 30.5
  dimension "d81" = 26.4
  dimension "d82" = 3
  dimension "d83" = 3
  dimension "d84" = 3
  dimension "d85" = 3
  dimension "d89" = 0.3
  dimension "d90" = 0.3
  dimension "d91" = 0.3
  dimension "d92" = 0.3
  constraints: 12 end point, 8 centre point, 4 coincident, 2 midpoint, 2 parallel, 1 horizontal, 1 perpendicular
  measures "d80" distance of L9.end L8.end
  measures "d81" distance of L8.end L7.end
  measures "d82" diameter of A0
  measures "d83" diameter of A1
  measures "d84" diameter of A2
  measures "d85" diameter of A3
  measures "d89" radial gap between concentric circles of A0 A4
  measures "d90" radial gap between concentric circles of A1 A5
  measures "d91" radial gap between concentric circles of A3 A6
  measures "d92" radial gap between concentric circles of A2 A7
extrude "Extrusion17" cut sketch "Sketch17" against normal up to surface (12.2 mm away)
sketch "Sketch18" plane through (0, 0, -6) normal (0, 0, -1) x (-1, 0, 0)
  line L0 (-39.8, 8) -> (-39.8, 4.3838) projected
  line L1 (-44.1838, 0) -> (-47.8, 0) projected
  line L2 (-47.8, 6) -> (-47.8, -39.8) projected
  circle A0 centre (-42.9, 3.1) radius 3 projected
  line L3 (-6.2, 4.9) -> (-72.3075, 4.9) projected
  line L4 (-39.7, 4.9) -> (-39.7, 0)
  line L5 (-72.3075, 0) -> (-10.2, 0) projected
  line L6 (-39.7, 4.9) -> (-47.9, 4.9)
  line L7 (-47.9, 4.9) -> (-47.9, -0.1)
  line L8 (-47.9, -0.1) -> (-39.7, -0.1)
  line L9 (-39.7, -0.1) -> (-39.7, 4.9)
  line L10 (-47.9, -0.1) -> (-55.9, -0.1)
  line L11 (-55.9, -0.1) -> (-55.9, 4.9)
  circle A1 centre (-52.7, 3.1) radius 1.1933 projected
  circle A2 centre (-52.7, 3.1) radius 1.4 projected
  circle A3 centre (-52.7, 3.1) radius 1.6 projected
  circle A4 centre (-52.7, 3.1) radius 1.5 projected
  circle A5 centre (-52.7, 3.1) radius 2.75 projected
  circle A6 centre (-52.7, 3.1) radius 1.4 projected
  point P0 (0, 0)
  dimension "d95" = 0.1
  dimension "d97" = 0.1
  dimension "d98" = 0.1
  dimension "d107" = 3.2
  constraints: 14 end point, 3 point on line, 2 horizontal, 2 parallel, 2 perpendicular, 1 vertical
  measures "d95" distance between parallel lines of L4 L0
  measures "d97" distance between parallel lines of L5 L8
  measures "d98" distance between parallel lines of L7 L2
  measures "d107" distance from line of L11 A3.centre
extrude "Extrusion18" cut sketch "Sketch18" against normal up to surface (6 mm away) contours L5 L9 L8 L2 L1 | L1 L2 L3 A0 L4 L5 | L5 L7 L3 L2 | L2 L8 L7 L5 | L7 L10 L11 L5 | L5 L11 L3 A5 L7 | L3 A0 | A5 L3 | L3 A5 | A1 | A2 | A3 | A4 picked at (-42.9851, 3.3036)
sketch "Sketch19" plane through (0, 0, -6) normal (0, 0, -1) x (-1, 0, 0)
  line L0 (-42.386, 1.7978) -> (-44.1838, 0) projected
  line L1 (-39.8, 4.3838) -> (-41.5978, 2.586) projected
  line L2 (-47.8, 6) -> (-47.8, -39.8) projected
  line L3 (-72.3075, 0) -> (-10.2, 0) projected
  line L4 (-39.7, 0) -> (-39.7, 4.9) projected
  line L5 (-44.1019, -0.0818) -> (-47.9, -0.0818)
  line L6 (-47.9, -0.0818) -> (-47.9, 0)
  line L7 (-54.7, 0) -> (-39.7, 0)
  line L8 (-39.7, 0) -> (-39.7, -3)
  line L9 (-39.7, -3) -> (-54.7, -3)
  line L10 (-54.7, -3) -> (-54.7, 0)
  line L11 (-39.7, -3) -> (-36.7, 0)
  line L12 (-39.7, -3) -> (-35.4574, -3) construction
  line L13 (-39.7, 0) -> (-36.7, 0)
  line L14 (-39.7, 0) -> (-10.2, 0) projected
  line L15 (-54.7, -3) -> (-57.7, 0)
  line L16 (-54.7, -3) -> (-50.4574, -3) construction
  line L17 (-57.7, 0) -> (-54.7, 0)
  line L18 (-47.9, -0.0818) -> (-51.4981, -0.0818)
  line L19 (-55.9, 4.9) -> (-55.9, 0) projected
  line L20 (-55.9, 4.3201) -> (-55.9, 0)
  line L21 (-57.7, 0) -> (-55.9, 0)
  line L22 (-39.7, 4.3201) -> (-41.3623, 2.6578)
  line L23 (-42.4578, 1.5623) -> (-44.1019, -0.0818)
  line L24 (-51.4981, -0.0818) -> (-53.1422, 1.5623)
  line L25 (-54.2377, 2.6578) -> (-55.9, 4.3201)
  line L26 (-41.3623, 2.6578) -> (-42.4578, 1.5623)
  line L27 (-53.1422, 1.5623) -> (-54.2377, 2.6578)
  point P0 (0, 0)
  dimension "d101" = 15
  dimension "d102" = 3
  dimension "d103" = 45
  dimension "d106" = 135
  dimension "d112" = 0
  constraints: 42 end point, 5 perpendicular, 5 point on line, 4 horizontal, 3 collinear, 3 parallel, 2 equal length
  measures "d101" distance of L8.end L9.end
  measures "d102" distance of L4.start L8.end
  measures "d103" angle of L12 L11
  measures "d106" angle of L16 L15
  measures "d112" vertical distance of L25.end L22.start
extrude "Extrusion19" add sketch "Sketch19" against normal up to surface (6 mm away) contours L5 L23 L3 L8 L9 L2 | L2 L9 L10 L3 L24 L18 L5 | L3 L19 L25 L27 L24 | L23 L26 L22 L4 L3 | L8 L3 L11 | L15 L3 L10
ref_plane "Work Plane8" through (72.3075, -16.9, -6) normal (0, 1, 0) x (1, 0, 0)
mirror "Mirror2" about plane through (72.3075, -16.9, -6) normal (0, 1, 0) of "Extrusion18", "Extrusion19"
sketch "Sketch20" plane through (72.3075, -16.9, -6) normal (0, 1, 0) x (1, 0, 0)
  line L0 (-26.3075, -6) -> (-26.3075, 0) projected
  line L1 (-16.3075, -6) -> (-16.3075, 0) projected
  line L2 (-16.3075, -6) -> (-26.3075, -6)
  line L3 (-26.3075, -6) -> (-26.3075, 0)
  line L4 (-26.3075, 0) -> (-16.3075, 0)
  line L5 (-16.3075, 0) -> (-16.3075, -6)
  line L6 (-30.3075, -6) -> (-30.3075, -0.5) projected
  line L7 (-26.3075, -6) -> (-30.3075, -0.5)
  line L8 (-30.3075, -6) -> (-26.3075, -6)
  line L9 (-26.3075, -6) -> (-26.3075, -0.5)
  line L10 (-26.3075, -0.5) -> (-30.3075, -0.5)
  line L11 (-30.3075, -0.5) -> (-30.3075, -6)
  point P0 (-72.3075, -6)
  constraints: 18 end point, 4 parallel, 2 horizontal, 2 perpendicular, 1 point on line
extrude "Extrusion20" cut sketch "Sketch20" along normal mid plane 28
sketch "Sketch21" plane through (72.3075, -16.9, -6) normal (0, 1, 0) x (1, 0, 0)
  circle A0 centre (-4.4945, -3) radius 1.45 projected
  line L0 (-16.3075, -6) -> (-1.3075, -6) projected
  line L1 (-16.3075, -6) -> (-16.3075, 0) projected
  line L2 (-16.3075, 0) -> (-1.3075, 0) projected
  line L3 (-1.3075, 0) -> (-1.3075, -6) projected
  line L4 (-26.3075, -0.5) -> (-30.3075, -0.5) projected
  line L5 (-30.3075, -0.5) -> (-30.3075, -6) projected
  line L6 (-30.3075, -6) -> (-35.7961, -6) projected
  line L7 (-35.7961, -6) -> (-35.7961, 0) projected
  line L8 (-35.7961, 0) -> (-26.3075, 0) projected
  line L9 (-26.3075, -0.5) -> (-26.3075, 0) projected
  line L10 (-11.3075, -1.636) -> (-11.3075, 0) projected
  line L11 (-16.3075, 0) -> (-11.3075, 0)
  line L12 (-11.3075, 0) -> (-11.3075, 5)
  line L13 (-11.3075, 5) -> (-16.3075, 5)
  line L14 (-16.3075, 5) -> (-16.3075, 0)
  line L15 (-29.8497, 0) -> (-30.9452, 0) projected
  line L16 (-16.3075, 5) -> (-30.3974, 5)
  line L17 (-30.3974, 5) -> (-30.3974, 0)
  line L18 (-30.3974, 0) -> (-16.3075, 0)
  line L19 (-16.3075, 0) -> (-16.3075, 5)
  point P0 (-72.3075, -6)
  dimension "d116" = 5
  constraints: 16 end point, 4 parallel, 2 horizontal, 2 perpendicular, 1 midpoint
  measures "d116" distance of L12.end L11.end
extrude "Extrusion21" add sketch "Sketch21" along normal mid plane 14 contours L14 L13 L12 L2 | L18 L8 L17 L16 L14
sketch "Sketch22" plane through (0, 0, -6) normal (0, 0, -1) x (-1, 0, 0)
  line L0 (-42, -12.2664) -> (-42, -6.1887) projected
  line L1 (-42, -12.2664) -> (-42, -6.1887) projected
  line L2 (-42, -6.1887) -> (-36.5113, -0.7) projected
  line L3 (-36.5113, -0.7) -> (-11, -0.7) projected
  line L4 (-11, -0.7) -> (-11, -4.3971) projected
  line L5 (-11, -4.3971) -> (-15.6532, -4.3971) projected
  arc A0 (-15.6532, -4.3971) -> (-30.5468, -4.3971) centre (-23.1, -16.9) ccw projected
  line L6 (-30.5468, -4.3971) -> (-34.1307, -4.3971) projected
  line L7 (-34.1307, -4.3971) -> (-42, -12.2664) projected
  line L8 (-42, -27.6113) -> (-42, -21.5336) projected
  line L9 (-34.1307, -29.4029) -> (-42, -21.5336) projected
  line L10 (-30.5468, -29.4029) -> (-34.1307, -29.4029) projected
  arc A1 (-30.5468, -29.4029) -> (-15.6532, -29.4029) centre (-23.1, -16.9) ccw projected
  line L11 (-11, -29.4029) -> (-15.6532, -29.4029) projected
  line L12 (-11, -33.1) -> (-11, -29.4029) projected
  line L13 (-36.5113, -33.1) -> (-11, -33.1) projected
  line L14 (-42, -27.6113) -> (-36.5113, -33.1) projected
  line L15 (-36.5113, -0.7) -> (-34.1307, -4.3971)
  line L16 (-34.1307, -29.4029) -> (-36.5113, -33.1)
  line L17 (-40.7, -10.9664) -> (-42, -12.2664) projected
  line L18 (-40.7, -10.9664) -> (-40.7, -12.2681) projected
  line L19 (-40.7, -21.5319) -> (-40.7, -12.2681) projected
  line L20 (-40.7, -22.8336) -> (-40.7, -21.5319) projected
  line L21 (-42, -21.5336) -> (-40.7, -22.8336) projected
  line L22 (-42, -27.6113) -> (-42, -21.5336) projected
  line L23 (-46, -23.6113) -> (-42, -27.6113) projected
  line L24 (-46, -10.1887) -> (-46, -23.6113) projected
  line L25 (-42, -6.1887) -> (-46, -10.1887) projected
  line L26 (-42, -12.2664) -> (-42, -6.1887) projected
  point P0 (0, 0)
  constraints: 4 end point
extrude "Extrusion22" add sketch "Sketch22" along normal blind 5 contours L7 L18 L19 L20 L9 L8 L23 L24 L25 L0 | L0 L2 L15 L7 | L8 L9 L16 L14
sketch "Sketch23" plane through (61, -9.9, -11) normal (0, 0, -1) x (-1, 0, 0)
  line L0 (19, -2.3664) -> (20.3, -1.0664) projected
  line L1 (19, -11.6336) -> (19, -2.3664) projected
  line L2 (20.3, -12.9336) -> (19, -11.6336) projected
  line L3 (20.3, -11.6319) -> (20.3, -12.9336) projected
  line L4 (20.3, -2.3681) -> (20.3, -11.6319) projected
  line L5 (20.3, -2.3681) -> (20.3, -1.0664) projected
  point P0 (61, 9.9)
extrude "Extrusion23" cut sketch "Sketch23" against normal blind 8
sketch "Sketch24" plane through (0, 0, -6) normal (0, 0, 1) x (1, 0, 0)
  line L0 (42, -12.2664) -> (40.7, -10.9664) projected
  line L1 (42, -21.5336) -> (42, -12.2664) projected
  line L2 (40.7, -22.8336) -> (42, -21.5336) projected
  line L3 (40.7, -21.5319) -> (40.7, -22.8336) projected
  line L4 (40.7, -12.2681) -> (40.7, -21.5319) projected
  line L5 (40.7, -12.2681) -> (40.7, -10.9664) projected
  point P0 (0, 0)
extrude "Extrusion24" add sketch "Sketch24" along normal up to surface (0.5 mm away)
chamfer "Chamfer1" distance 4 angle 45 3 edges at (42, -9.2275, 0) (42, -24.5725, 0) (40.7, -16.9, 0)
chamfer "Chamfer2" distance 5.5 angle 45 2 edges at (11, -2.5486, 0) (11, -31.2514, 0)
sketch "Sketch27" plane through (0, 0, 0) normal (0, 0, 1) x (1, 0, 0)
  arc A0 (77.0649, 0) -> (74.5351, 0) centre (75.8, 0.6) ccw construction
  arc A1 (74.5351, -33.8) -> (77.0649, -33.8) centre (75.8, -34.4) ccw construction
  line L0 (57.7, -33.8) -> (74.5351, -33.8) construction
  line L1 (57.7, -33.8) -> (54.8, -30.9) construction
  line L2 (54.8, -30.9) -> (42, -30.9) construction
  line L3 (42, -30.9) -> (42, -30.8) construction
  line L4 (42, -30.8) -> (39.7, -30.8) construction
  line L5 (39.7, -30.8) -> (36.7, -33.8) construction
  line L6 (10.2, -33.8) -> (36.7, -33.8) construction
  line L7 (10.2, -29.4029) -> (10.2, -33.8) construction
  arc A2 (10.2, -4.3971) -> (10.2, -29.4029) centre (14.0958, -16.9) ccw construction
  line L8 (10.2, -4.3971) -> (10.2, 0) construction
  line L9 (10.2, 0) -> (36.7, 0) construction
  line L10 (39.7, -3) -> (36.7, 0) construction
  line L11 (42, -3) -> (39.7, -3) construction
  line L12 (42, -3) -> (42, -2.9) construction
  line L13 (42, -2.9) -> (54.8, -2.9) construction
  line L14 (57.7, 0) -> (54.8, -2.9) construction
  line L15 (57.7, 0) -> (74.5351, 0) construction
  line L16 (89.6, 4.9) -> (55.9, 4.9) construction
  line L17 (55.9, 4.9) -> (55.9, 4.3201) construction
  line L18 (51.4981, -0.0818) -> (55.9, 4.3201) construction
  line L19 (44.1019, -0.0818) -> (51.4981, -0.0818) construction
  line L20 (39.7, 4.3201) -> (44.1019, -0.0818) construction
  line L21 (39.7, 4.3201) -> (39.7, 4.9) construction
  line L22 (39.7, 4.9) -> (6.2, 4.9) construction
  line L23 (6.2, 4.9) -> (6.2, -0.2) construction
  line L24 (6.2, -0.2) -> (-2, -0.2) construction
  line L25 (-2, -0.2) -> (-2, -33.6) construction
  line L26 (6.2, -33.6) -> (-2, -33.6) construction
  line L27 (6.2, -38.7) -> (6.2, -33.6) construction
  line L28 (39.7, -38.7) -> (6.2, -38.7) construction
  line L29 (39.7, -38.7) -> (39.7, -38.1201) construction
  line L30 (39.7, -38.1201) -> (44.1019, -33.7182) construction
  line L31 (44.1019, -33.7182) -> (51.4981, -33.7182) construction
  line L32 (51.4981, -33.7182) -> (55.9, -38.1201) construction
  line L33 (55.9, -38.1201) -> (55.9, -38.7) construction
  line L34 (89.6, -38.7) -> (55.9, -38.7) construction
  line L35 (16.5, -3.9301) -> (16.5, -0.7) construction
  arc A3 (30.5468, -4.3971) -> (16.5, -3.9301) centre (23.1, -16.9) ccw construction
  line L36 (30.5468, -4.3971) -> (34.1307, -4.3971) construction
  line L37 (34.1307, -4.3971) -> (38, -8.2664) construction
  line L38 (38, -2.1887) -> (38, -8.2664) construction
  line L39 (38, -2.1887) -> (36.5113, -0.7) construction
  line L40 (36.5113, -0.7) -> (16.5, -0.7) construction
  line L41 (16.5, -33.1) -> (16.5, -29.8699) construction
  line L42 (36.5113, -33.1) -> (16.5, -33.1) construction
  line L43 (38, -31.6113) -> (36.5113, -33.1) construction
  line L44 (38, -25.5336) -> (38, -31.6113) construction
  line L45 (34.1307, -29.4029) -> (38, -25.5336) construction
  line L46 (30.5468, -29.4029) -> (34.1307, -29.4029) construction
  arc A4 (16.5, -29.8699) -> (30.5468, -29.4029) centre (23.1, -16.9) ccw construction
  line L47 (10.2, -33.1) -> (36.5113, -33.1) projected
  line L48 (36.5113, -33.1) -> (10.2, -33.1)
  line L49 (10.2, -29.4029) -> (10.2, -33.1) projected
  line L50 (10.2, -32.95) -> (36.6613, -32.95)
  line L51 (36.5113, -33.1) -> (46, -23.6113) projected
  line L52 (10.2, -32.95) -> (10.2, -33.1)
  line L53 (36.5113, -33.1) -> (36.6613, -32.95)
  line L54 (-21.96, -16.9) -> (117.76, -16.9) construction
  line L55 (36.5113, -0.7) -> (16.5, -0.7) construction
  line L56 (10.2, -0.7) -> (36.5113, -0.7)
  line L57 (36.5113, -0.7) -> (10.2, -0.7)
  line L58 (10.2, -0.85) -> (36.6613, -0.85)
  line L59 (10.2, -0.85) -> (10.2, -0.7)
  line L60 (36.5113, -0.7) -> (36.6613, -0.85)
  line L61 (77.0649, -33.8) -> (85.8, -33.8) projected
  line L62 (77.0649, 0) -> (85.8, 0) projected
  line L63 (85.8, 0) -> (85.8, -4.2) projected
  line L64 (85.8, -4.2) -> (94.1838, -4.2) projected
  line L65 (94.1838, -4.2) -> (94.1838, -29.6) projected
  line L66 (85.8, -29.6) -> (94.1838, -29.6) projected
  line L67 (85.8, -33.8) -> (85.8, -29.6) projected
  line L68 (89.6, -33.6) -> (89.6, -38.7) projected
  line L69 (97.8, -33.6) -> (89.6, -33.6) projected
  line L70 (97.8, -33.6) -> (97.8, -0.2) projected
  line L71 (97.8, -0.2) -> (89.6, -0.2) projected
  line L72 (89.6, -0.2) -> (89.6, 4.9) projected
  point P0 (0, 0)
  dimension "d141" = 0.15
  constraints: 20 end point, 3 symmetric about line, 2 collinear, 2 point on line, 1 horizontal, 1 parallel
  measures "d141" distance between parallel lines of L42 L50
extrude "Extrusion27" cut sketch "Sketch27" against normal through all
sketch "Sketch28" plane through (0, 0, 0) normal (0, 0, 1) x (1, 0, 0)
  line L0 (36.6613, -0.85) -> (16.5, -0.85) construction
  line L1 (16.5, -3.9301) -> (16.5, -0.85) construction
  arc A0 (30.5468, -4.3971) -> (16.5, -3.9301) centre (23.1, -16.9) ccw construction
  line L2 (30.5468, -4.3971) -> (34.1307, -4.3971) construction
  line L3 (34.1307, -4.3971) -> (38, -8.2664) construction
  line L4 (38, -2.1887) -> (38, -8.2664) construction
  line L5 (38, -2.1887) -> (36.6613, -0.85) construction
  line L6 (42, -6.1887) -> (38, -2.1887) construction
  line L7 (38, -2.1887) -> (38, -8.2664) construction
  line L8 (38, -8.2664) -> (42, -12.2664) construction
  line L9 (42, -12.2664) -> (42, -6.1887) construction
  line L10 (34.1307, -29.4029) -> (36.4148, -32.95) construction
  line L11 (16.5, -32.95) -> (36.6613, -32.95) construction
  line L12 (38, -31.6113) -> (36.6613, -32.95) construction
  line L13 (38, -25.5336) -> (38, -31.6113) construction
  line L14 (34.1307, -29.4029) -> (38, -25.5336) construction
  line L15 (30.5468, -29.4029) -> (34.1307, -29.4029) construction
  arc A1 (16.5, -29.8699) -> (30.5468, -29.4029) centre (23.1, -16.9) ccw construction
  line L16 (16.5, -32.95) -> (16.5, -29.8699) construction
  line L17 (42, -21.5336) -> (38, -25.5336) construction
  line L18 (38, -25.5336) -> (38, -31.6113) construction
  line L19 (38, -31.6113) -> (42, -27.6113) construction
  line L20 (42, -27.6113) -> (42, -21.5336) construction
  line L21 (36.6613, -32.95) -> (42, -27.6113)
  line L22 (16.5, -32.95) -> (36.6613, -32.95) projected
  line L23 (36.4492, -32.95) -> (42, -27.3992)
  line L24 (36.4492, -32.95) -> (36.6613, -32.95)
  line L25 (46, -23.6113) -> (42, -27.6113) projected
  line L26 (42, -27.3992) -> (42, -27.6113)
  line L27 (-21.96, -16.9) -> (117.76, -16.9) construction
  line L28 (36.6613, -0.85) -> (42, -6.1887)
  line L29 (36.4492, -0.85) -> (42, -6.4008)
  line L30 (36.4492, -0.85) -> (36.6613, -0.85)
  line L31 (42, -6.4008) -> (42, -6.1887)
  point P0 (0, 0)
  point P1 (36.4148, -0.85)
  dimension "d144" = 0.15
  constraints: 16 end point, 3 symmetric about line, 2 point on line, 1 collinear, 1 horizontal, 1 parallel, 1 vertical
  measures "d144" distance between parallel lines of L19 L23
extrude "Extrusion28" cut sketch "Sketch28" against normal up to surface (11 mm away)